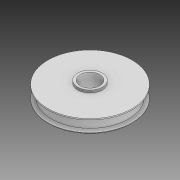
# Autodesk Inventor part: DrivenPulley
Saved by Autodesk Inventor 2020 (Build 240168000, 168)
## iProperties
Created: 2021-05-16
Part Number: DrivenPulley
Material: Generic
Document SubType Name: Modeling
Designer: DDeGo
Density: 1 g/cm^3
Appearance: Default
Author: DDeGo
Autodesk Inventor part; units mm, degrees
ref_plane "XZ Plane" through (0, 0, 0) normal (0, 1, 0) x (-1, 0, 0)
ref_plane "XY Plane" through (0, 0, 0) normal (0, 0, 1) x (1, 0, 0)
sketch "Sketch1" plane through (0, 0, 0) normal (0, 0, 1) x (1, 0, 0)
  line L0 (0, 0) -> (0, 16.1) construction
  line L1 (0, 0) -> (4.1, 0) construction
  line L2 (4.1, 0) -> (4.1, 16.1)
  line L3 (4.1, 16.1) -> (0, 16.1) construction
  line L4 (4.1, 16.1) -> (17.5, 16.1) construction
  line L5 (17.5, 16.1) -> (17.5, 15.6)
  line L6 (17.5, 15.6) -> (16, 15.1)
  line L7 (16, 15.1) -> (16, 11.5)
  line L8 (16, 11.5) -> (17.5, 11)
  line L9 (17.5, 11) -> (17.5, 10)
  line L10 (17.5, 10) -> (9, 6)
  line L11 (9, 6) -> (9, 0)
  line L12 (9, 0) -> (4.1, 0)
  line L13 (9, 0) -> (5.1, -1) construction
  line L14 (5.1, -1) -> (4.1, -1) construction
  line L15 (4.1, -1) -> (4.1, 0) construction
  line L16 (4.1, 16.1) -> (4.1, 16.6)
  line L17 (4.1, 16.6) -> (5.1, 16.6) construction
  line L18 (5.1, 16.6) -> (17.5, 16.1)
  line L19 (5.1, 16.6) -> (5.1, 17.6)
  line L20 (5.1, 17.6) -> (4.1, 17.6)
  line L21 (4.1, 17.6) -> (4.1, 16.6)
  dimension "d0" = 4.1
  dimension "d1" = 3.6
  dimension "d2" = 0.5
  dimension "d3" = 1
  dimension "d4" = 0.5
  dimension "d5" = 1.5
  dimension "d6" = 9
  dimension "d7" = 16
  dimension "d8" = 4
  dimension "d9" = 6
  dimension "d11" = 1
  dimension "d12" = 1
  dimension "d13" = 1
  dimension "d14" = 0.5
  dimension "d15" = 1
  constraints: 44 end point, 7 perpendicular, 4 point on line, 3 vertical, 2 horizontal, 2 parallel, 1 equal length
  measures "d0" distance between parallel lines of L2 L0
  measures "d1" distance of L6.end L7.end
  measures "d2" distance of L4.end L5.end
  measures "d3" distance of L8.end L9.end
  measures "d4" vertical distance of L7.end L8.end
  measures "d5" distance between parallel lines of L7 L9
  measures "d6" distance between parallel lines of L0 L11
  measures "d7" distance between parallel lines of L0 L7
  measures "d8" vertical distance of L9.end L10.end
  measures "d9" distance of L10.end L11.end
  measures "d11" distance of L13.end L14.end
  measures "d12" distance between parallel lines of L12 L14
  measures "d13" distance of L16.end L17.end
  measures "d14" distance of L2.end L16.end
  measures "d15" distance of L20.end L16.end
revolve "Revolution1" add sketch "Sketch1" angle 360 about axis through (0, 0, 0) along (0, 1, 0)
ref_plane "Work Plane1" through (4, 0, 0) normal (1, 0, 0) x (0, 1, 0)
sketch "Sketch2" plane through (4, 0, 0) normal (1, 0, 0) x (0, 1, 0)
  line L0 (0, 0) -> (2.85, 0) construction
  line L1 (0, 2.85) -> (5.7, 2.85)
  line L2 (5.7, 2.85) -> (5.7, -2.85)
  line L3 (5.7, -2.85) -> (0, -2.85)
  line L4 (0, -2.85) -> (0, 2.85)
  line L5 (0, 2.85) -> (5.7, -2.85) construction
  line L6 (5.7, 2.85) -> (0, -2.85) construction
  line L7 (0, 4.1) -> (0, -4.1) projected
  dimension "d17" = 5.7
  dimension "d18" = 5.7
  constraints: 14 end point, 2 horizontal, 2 midpoint, 2 parallel, 1 perpendicular, 1 point on line
  measures "d17" distance of L1.end L2.end
  measures "d18" distance of L2.end L3.end
extrude "Extrusion1" cut sketch "Sketch2" along normal blind 2.5 and the other way blind 3
sketch "Sketch3" plane through (4, 0, 0) normal (1, 0, 0) x (0, 1, 0)
  line L0 (5.7, -2.85) -> (0, 2.85) construction
  circle A0 centre (2.85, 0) radius 1.7
  point P0 (0, 0)
  dimension "d23" = 3.4
  constraints: 2 end point, 1 centre point, 1 midpoint
  measures "d23" diameter of A0
extrude "Extrusion2" cut sketch "Sketch3" along normal through all
sketch "Sketch4" plane through (0, 0, 0) normal (0, -1, 0) x (1, 0, 0)
  circle A0 centre (0, 0) radius 26.9979
  constraints: 1 centre point, 1 coincident
extrude "SetScrewDelete" cut sketch "Sketch4" against normal blind 10.5
chamfer "Chamfer1" distance 0.3 angle 45 1 edges at (-17.5, 10.5, 0)
body "Solid1"
